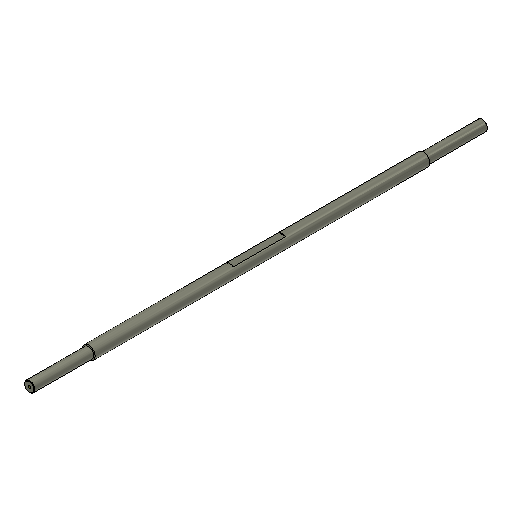
# Autodesk Inventor part: TL20240701-10110CV-007
Saved by Autodesk Inventor 2022.5 (Build 265521000, 521)
## iProperties
Category: DRIVE UNIT ASSY
Manager: 호상태
Company: 현대 트랜시스(대유)
Created: 2023-01-19
Part Number: TL20240701-10110CV-007
Project: SW PJT
Checked By: 김형민
Engr Approved By: 김시현
Material: S45C
Description: 0
Document SubType Name: Modeling
Mfg Approved By: 호상태
Designer: 박성규
Density: 7.87 g/cm^3
Appearance: Plating Kanizen
User Status: 1 x18
Stock Number: 007
DETAIL: Coveryor Assembly
M/C TITLE: MEa/NEa차종 시트조립라인
PARTS NAME: Bracket
SPECIFICATION: TA20221101-CV200000-015
DocNumber: 221118_Standard_v1
Folder: .\
VDS_Category: 엔지니어링
Detail Description: Processed products
Title: SHAFT
Subject: SW차종 시트조립라인
Author: 박성규
Revision Number: A
Autodesk Inventor part; units mm, degrees
ref_plane "YZ Plane" through (0, 0, 0) normal (1, 0, 0) x (0, 1, 0)
sketch "스케치11" plane through (0, 0, 0) normal (0, 0, 1) x (1, 0, 0)
  circle A0 centre (0, 0) radius 10
  dimension "d60" = 20
  constraints: 1 centre point, 1 coincident
  measures "d60" diameter of A0
extrude "돌출4" add sketch "스케치11" along normal mid plane 864.6
sketch "스케치16" plane through (0, 0, 0) normal (0, 0, 1) x (1, 0, 0)
  circle A0 centre (0, 0) radius 12.5
  dimension "d94" = 25
  constraints: 1 centre point, 1 coincident
  measures "d94" diameter of A0
extrude "돌출7" add sketch "스케치16" along normal mid plane 638
ref_plane "작업 평면1" through (0, 0, -354) normal (0, 0, -1) x (-1, 0, 0)
ref_plane "작업 평면2" through (0, 0, 344) normal (0, 0, 1) x (1, 0, 0)
sketch "스케치12" plane through (0, 0, -354) normal (0, 0, -1) x (-1, 0, 0)
  line L0 (-3, -6.5) -> (3, -6.5)
  line L1 (3, -6.5) -> (3, -12.5)
  line L2 (3, -12.5) -> (-3, -12.5)
  line L3 (-3, -12.5) -> (-3, -6.5)
  line L4 (-3, -6.5) -> (3, -12.5) construction
  line L5 (3, -6.5) -> (-3, -12.5) construction
  point P0 (0, 0)
  point P1 (0, -9.5)
  point P2 (0, -9.5)
  dimension "d65" = 6
  dimension "d66" = 6
  dimension "d67" = 6.5
  constraints: 12 end point, 3 midpoint, 2 parallel, 1 horizontal, 1 perpendicular, 1 vertical alignment
  measures "d65" distance of L1.end L2.end
  measures "d66" distance of L0.end L1.end
  measures "d67" distance from line of point (0, 0) L0
extrude "돌출5" cut sketch "스케치12" along normal mid plane 68
sketch "스케치13" plane through (0, 0, 344) normal (0, 0, 1) x (1, 0, 0)
  line L0 (-3, -6.5) -> (3, -6.5)
  line L1 (3, -6.5) -> (3, -12.5)
  line L2 (3, -12.5) -> (-3, -12.5)
  line L3 (-3, -12.5) -> (-3, -6.5)
  line L4 (-3, -6.5) -> (3, -12.5) construction
  line L5 (3, -6.5) -> (-3, -12.5) construction
  point P0 (0, 0)
  point P1 (0, -9.5)
  point P2 (0, -9.5)
  dimension "d70" = 6
  dimension "d71" = 6
  dimension "d72" = 6.5
  constraints: 12 end point, 3 midpoint, 2 parallel, 1 horizontal, 1 perpendicular, 1 vertical alignment
  measures "d70" distance of L0.end L1.end
  measures "d71" distance of L1.end L2.end
  measures "d72" distance from line of point (0, 0) L0
extrude "돌출6" cut sketch "스케치13" along normal mid plane 48
fillet "모깎기2" radius 3 4 edges at (3, -8.0197, -320) (-3, -8.0197, -320) (-3, -8.0197, -388) (3, -8.0197, -388)
fillet "모깎기3" radius 3 4 edges at (-3, -8.0197, 320) (3, -8.0197, 320) (3, -8.0197, 368) (-3, -8.0197, 368)
sketch "스케치14" plane through (0, 0, -432.3) normal (0, 0, -1) x (-1, 0, 0)
  circle A0 centre (0, 0) radius 10 construction
  constraints: 1 coincident
hole "구멍5" at (0, 0, -432.3) direction (0, 0, 1) diameter 4.917 depth 17.1 tip angle 118 thread size "M6x1" class "6H" standard "ISO Metric profile"
sketch "스케치15" plane through (0, 0, 432.3) normal (0, 0, 1) x (1, 0, 0)
  circle A0 centre (0, 0) radius 10 construction
  constraints: 1 coincident
hole "구멍6" at (0, 0, 432.3) direction (0, 0, -1) diameter 4.917 depth 17.1 tip angle 118 thread size "M6x1" class "6H" standard "ISO Metric profile"
chamfer "모따기1" distance 1 angle 45 2 edges at (-10, 0, 432.3) (-10, 0, -432.3)
sketch "스케치17" plane through (0, 0, 0) normal (0, 0, 1) x (1, 0, 0)
  line L0 (-10, 20.5) -> (10, 20.5)
  line L1 (10, 20.5) -> (10, 10.5)
  line L2 (10, 10.5) -> (-10, 10.5)
  line L3 (-10, 10.5) -> (-10, 20.5)
  line L4 (-10, -10.5) -> (10, -10.5)
  line L5 (10, -10.5) -> (10, -20.5)
  line L6 (10, -20.5) -> (-10, -20.5)
  line L7 (-10, -20.5) -> (-10, -10.5)
  point P0 (0, 0)
  point P1 (0, 20.5)
  point P2 (0, -20.5)
  dimension "d99" = 10.5
  dimension "d100" = 10.5
  dimension "d101" = 10
  dimension "d102" = 20
  constraints: 16 end point, 4 parallel, 2 equal length, 2 horizontal, 2 midpoint, 2 perpendicular, 2 vertical alignment
  measures "d99" distance from line of point (0, 0) L2
  measures "d100" distance from line of point (0, 0) L4
  measures "d101" distance of L0.end L1.end
  measures "d102" distance of L0.start L0.end
extrude "돌출8" cut sketch "스케치17" along normal mid plane 100
